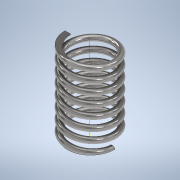
# Autodesk Inventor part: spring
Saved by Autodesk Inventor 2022 (Build 260153000, 153)
## iProperties
Created: 2021-07-30
Part Number: spring
Material: Steel, High Strength, Low Alloy
Document SubType Name: Modeling
Designer: Ian Kibandi
Density: 7.85 g/cm^3
Appearance: Steel - Polished
Author: Ian Kibandi
Autodesk Inventor part; units mm, degrees
ref_plane "YZ Plane" through (0, 0, 0) normal (1, 0, 0) x (0, 1, 0)
ref_plane "XZ Plane" through (0, 0, 0) normal (0, 1, 0) x (-1, 0, 0)
ref_plane "XY Plane" through (0, 0, 0) normal (0, 0, 1) x (1, 0, 0)
sketch "Sketch1" plane through (0, 0, 0) normal (0, 1, 0) x (-1, 0, 0)
  point P0 (0, 0)
sketch "Sketch2" plane through (0, 0, 0) normal (0, 1, 0) x (-1, 0, 0)
  circle A0 centre (0, 0) radius 45
  dimension "d0" = 90
  constraints: 1 centre point, 1 coincident
  measures "d0" diameter of A0
extrude "Extrusion1" add sketch "Sketch2" along normal blind 140
sketch "Sketch3" plane through (0, 0, 0) normal (0, 0, 1) x (1, 0, 0)
  line L0 (45, 140) -> (-45, 140) projected
  circle A0 centre (-40, 140) radius 5
  point P0 (0, 0)
  dimension "d28" = 10
  constraints: 1 centre point, 1 point on line
  measures "d28" diameter of A0
coil "Coil3" sketch "Sketch3" operation intersect axis through (0, 0, 0) along (0, -1, 0) pitch 18.8 turns 7.5 hand left
body "Solid1"
